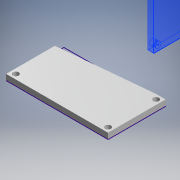
# Autodesk Inventor part: head-sideplate
Saved by Autodesk Inventor 2016 (Build 200138000, 138)
## iProperties
Created: 2015-04-29
Part Number: head-sideplate
Material: Aluminum 6061
Document SubType Name: Modeling
Designer: ax
Density: 2.7 g/cm^3
Appearance: Aluminum - Flat
Mass: 11.8036 g
Surface Area: 34.8403 cm^2
Volume: 4.37172 cm^3
Author: ax
Autodesk Inventor part; units mm, degrees
ref_plane "YZ Plane" through (0, 0, 0) normal (1, 0, 0) x (0, 1, 0)
ref_plane "XZ Plane" through (0, 0, 0) normal (0, 1, 0) x (-1, 0, 0)
ref_plane "XY Plane" through (0, 0, 0) normal (0, 0, 1) x (1, 0, 0)
sketch "Sketch1" plane through (0, 0, 0) normal (0, 0, 1) x (1, 0, 0)
  line L0 (0, 0) -> (53, 0)
  line L1 (53, 0) -> (53, 30)
  line L2 (53, 30) -> (0, 30)
  line L3 (0, 30) -> (0, 0)
  point P0 (2.5, 2.5)
  point P1 (50.5, 2.5)
  point P2 (50.5, 27.5)
  dimension "d0" = 53
  dimension "d1" = 30
  constraints: 8 end point, 2 parallel, 1 horizontal, 1 perpendicular
  measures "d0" distance of L2.end L1.end
  measures "d1" distance of L1.end L0.end
extrude "Extrusion1" add sketch "Sketch1" along normal blind 3
hole "Hole1" at (2.5, 2.5, 0) at (50.5, 2.5, 0) at (50.5, 27.5, 0) direction (0, 0, 1) diameter 3 end through all
sketch "Sketch2" plane through (0, 0, 3) normal (0, 0, 1) x (1, 0, 0)
  line L0 (53, 0) -> (53, 30) projected
  line L1 (53, 30) -> (48, 30)
  line L2 (53, 30) -> (0, 30) projected
  line L3 (48, 30) -> (0, 25.3519)
  line L4 (0, 30) -> (0, 0) projected
  line L5 (0, 30) -> (48, 30)
  dimension "d11" = 5
  constraints: 6 end point, 2 point on line, 1 collinear
  measures "d11" distance of L0.end L1.end
extrude "Extrusion2" cut sketch "Sketch2" against normal through all
body "Solid1"
